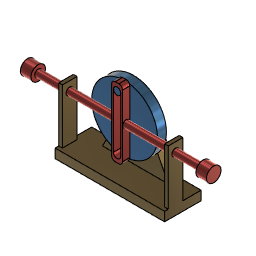
Scotch Yoke Mechanism (Autodesk Fusion 360 design; units mm, degrees)
Autodesk Fusion 360 part; units mm, degrees
sketch "Holder Base" plane through (0, 0, 0) normal (0, 0, 1) x (1, 0, 0)
  line L0 (150, -50) -> (-150, -50)
  line L1 (-150, -50) -> (-150, 50)
  line L2 (-150, 50) -> (150, 50)
  line L3 (150, 50) -> (150, -50)
  line L4 (150, -50) -> (-150, 50) construction
  line L5 (-150, -50) -> (150, 50) construction
  dimension "d1" = 300
  dimension "d2" = 100
  constraint horizontal L0
  constraint perpendicular L0 L1
  constraint parallel L0 L2
  constraint parallel L1 L3
  constraint coincident L4 origin
  constraint coincident L5 origin
  measures "d1" distance of L1.end L2.end
  measures "d2" distance of L0.end L1.end
extrude "Extrude1" add sketch "Holder Base" along normal blind 25 makes body 1
sketch "Holder" plane through (0, 0, 25) normal (0, 0, 1) x (-1, 0, 0)
  line L0 (-150, -50) -> (150, -50)
  line L1 (150, -50) -> (150, 50)
  line L2 (150, 50) -> (-150, 50)
  line L3 (-150, 50) -> (-150, -50)
  line L4 (-90, -50) -> (90, -50)
  line L5 (90, -50) -> (90, -20)
  line L6 (90, -20) -> (-90, -20)
  line L7 (-90, -20) -> (-90, -50)
  constraint horizontal L4
  constraint vertical L5
  constraint horizontal L6
  constraint vertical L7
  constraint coincident L0 L4.start
extrude "Extrude2" add sketch "Holder" along normal blind 150 contours L0 L4 L5 L6 L7 bodies 1
sketch "Holder Shape" plane through (0, 20, 0) normal (0, -1, 0) x (1, 0, 0)
  line L0 (-90, 25) -> (90, 25)
  line L1 (90, 25) -> (90, 175)
  line L2 (90, 175) -> (-90, 175)
  line L3 (-90, 175) -> (-90, 25)
  circle A0 centre (0, 150) radius 25
  line L4 (-90, 25) -> (-22.3903, 161.121)
  line L5 (90, 25) -> (22.3903, 161.121)
  circle A1 centre (0, 150) radius 10
  constraint tangent L2 A0
  constraint coincident L0.start L3.end
  constraint coincident A0 L4.end
  constraint tangent A0 L4
  constraint coincident L0.end L1.start
  constraint coincident A0 L5.end
  constraint tangent A0 L5
  constraint concentric A0 A1
extrude "Extrude3" cut sketch "Holder Shape" against normal blind 70 contours L2 L3 A0 L4 | L1 L2 A0 L5 bodies 1
sketch "Crank" plane through (0, 20, 93.0605) normal (0, -1, 0) x (1, 0, 0)
  circle A0 centre (0, 56.9395) radius 90
  point P0 (0, 56.9395)
  dimension "d9" = 180
  constraint coincident P0 A0.centre
  measures "d9" diameter of A0
extrude "Extrude4" add sketch "Crank" along normal blind 30 and the other way blind -10 separate body makes body 2
extrude "Extrude5" cut sketch "Holder Shape" along normal blind 150 contours A1 bodies 2
extrude "Extrude6" add sketch "Holder Shape" along normal blind 4.8 contours A0 bodies 1
extrude "Extrude7" add 1 faces at (62.9983, 10, 145.5287) along direction (0, 1, 0) blind 5 on bodies 2 bodies 2
extrude "Extrude8" add sketch "Holder Shape" along normal blind 40 contours A1 bodies 1
extrude "Extrude9" cut 1 faces at (3.0405, -20, 148.0569) along direction (0, 1, 0) blind 10 on bodies 1 bodies 1
move_face "OffsetFaces1" offset -0.3 1 faces at (9.9876, 6.6667, 150.4985) on bodies 2
move_face "OffsetFaces2" offset -0.3 1 faces at (10.2872, -1.6667, 149.4866) on bodies 2
sketch "Crank Pin" plane through (0, -10, 0) normal (0, -1, 0) x (1, 0, 0)
  circle A0 centre (75, 150) radius 10
extrude "Extrude10" add sketch "Crank Pin" along normal blind 20 bodies 2
sketch "Slotted Link" plane through (0, -10, 0) normal (0, -1, 0) x (1, 0, 0)
  line L0 (75, 235) -> (75, 235)
  line L1 (85, 225) -> (85, 75)
  line L2 (75, 65) -> (75, 65)
  line L3 (65, 75) -> (65, 225)
  line L4 (70, 245) -> (80, 245)
  line L5 (90, 235) -> (90, 64.9408)
  line L6 (80, 54.9408) -> (70, 54.9408)
  line L7 (60, 64.9408) -> (60, 235)
  arc A0 (85, 225) -> (75, 235) centre (75, 225) ccw
  arc A1 (75, 235) -> (65, 225) centre (75, 225) ccw
  arc A2 (90, 235) -> (80, 245) centre (80, 235) ccw
  arc A3 (70, 245) -> (60, 235) centre (70, 235) ccw
  arc A4 (80, 54.9408) -> (90, 64.9408) centre (80, 64.9408) ccw
  arc A5 (60, 64.9408) -> (70, 54.9408) centre (70, 64.9408) ccw
  arc A6 (75, 65) -> (85, 75) centre (75, 75) ccw
  arc A7 (65, 75) -> (75, 65) centre (75, 75) ccw
  dimension "d28" = 10
  dimension "d29" = 10
  dimension "d30" = 10
  dimension "d31" = 10
  constraint vertical L1
  constraint vertical L3
  constraint horizontal L4
  constraint vertical L5
  constraint horizontal L6
  constraint vertical L7
  constraint tangent L1 A0
  constraint tangent L3 A1
  constraint tangent L4 A2
  constraint tangent L5 A2
  constraint tangent L4 A3
  constraint tangent L7 A3
  constraint equal A2 A3
  constraint tangent L5 A4
  constraint tangent L6 A4
  constraint equal A2 A4
  constraint tangent L6 A5
  constraint tangent L7 A5
  constraint equal A2 A5
  constraint tangent L1 A6
  constraint equal A2 A6
  constraint tangent L3 A7
  measures "d28" radius of A0
  measures "d29" radius of A1
  measures "d30" radius of A2
  measures "d31" radius of A7
extrude "Extrude11" add sketch "Slotted Link" along normal blind 20 separate body makes body 3
extrude "Extrude12" cut 1 faces at (47.1382, -10, 124.9243) along direction (0, 1, 0) blind 0.3 on bodies 2 bodies 2
move_face "OffsetFaces3" offset -0.3 1 faces at (84.9876, -16.4667, 149.5015) on bodies 2
sketch "Piston Holders" plane through (0, 0, 25) normal (0, 0, 1) x (-1, 0, 0)
  line L0 (90, -20) -> (90, -50)
  line L1 (90, -50) -> (150, -50)
  line L2 (150, -50) -> (150, 50)
  line L3 (150, 50) -> (-150, 50)
  line L4 (-150, 50) -> (-150, -50)
  line L5 (-150, -50) -> (-90, -50)
  line L6 (-90, -50) -> (-90, -20)
  line L7 (-90, -20) -> (90, -20)
  line L8 (140, 0) -> (150, 0)
  line L9 (150, 0) -> (150, 40)
  line L10 (150, 40) -> (140, 40)
  line L11 (140, 40) -> (140, 0)
  line L12 (-150, 0) -> (-140, 0)
  line L13 (-140, 0) -> (-140, 40)
  line L14 (-140, 40) -> (-150, 40)
  line L15 (-150, 40) -> (-150, 0)
  constraint horizontal L8
  constraint vertical L9
  constraint horizontal L10
  constraint vertical L11
  constraint coincident L2 L9.end
  constraint horizontal L12
  constraint vertical L13
  constraint horizontal L14
  constraint vertical L15
  constraint midpoint L4 L12.start
extrude "Extrude13" add sketch "Piston Holders" along normal blind 150 contours L2 L8 L9 L10 L11 | L4 L12 L13 L14 L15 bodies 1
sketch "Right Piston" plane through (90, 0, 0) normal (1, 0, 0) x (0, 1, 0)
  line L0 (-10, 64.9408) -> (-10, 235)
  line L1 (-10, 235) -> (-30, 235)
  line L2 (-30, 235) -> (-30, 64.9408)
  line L3 (-30, 64.9408) -> (-10, 64.9408)
  circle A0 centre (-20, 150) radius 10
  constraint tangent L2 A0
sketch "Left Piston" plane through (60, 0, 0) normal (-1, 0, 0) x (0, -1, 0)
  line L0 (10, 235) -> (10, 64.9408)
  line L1 (10, 64.9408) -> (30, 64.9408)
  line L2 (30, 64.9408) -> (30, 235)
  line L3 (30, 235) -> (10, 235)
  circle A0 centre (20, 150) radius 10
extrude "Extrude14" cut sketch "Right Piston" along normal blind 75 contours A0 bodies 1
extrude "Extrude15" cut sketch "Left Piston" along normal blind 230 contours A0 bodies 1
extrude "Extrude16" add sketch "Left Piston" along normal blind 240 contours A0 bodies 3
extrude "Extrude17" add sketch "Right Piston" along normal blind 240 contours A0 bodies 3
sketch "Left Piston End" plane through (-180, 0, 0) normal (-1, 0, 0) x (0, -1, 0)
  circle A0 centre (20, 150) radius 10
  circle A1 centre (20, 150) radius 20
  constraint concentric A0 A1
extrude "Extrude18" add sketch "Left Piston End" against normal blind 29 bodies 3
sketch "Right Piston End" plane through (330, 0, 0) normal (1, 0, 0) x (0, 1, 0)
  circle A0 centre (-20, 150) radius 10
  circle A1 centre (-20, 150) radius 20
  dimension "d49" = 40
  constraint concentric A0 A1
  measures "d49" diameter of A1
extrude "Extrude19" add sketch "Right Piston End" against normal blind 29 bodies 3
move_face "OffsetFaces4" offset -0.3 2 faces at (160.3333, -10.0497, 149.0043) (-80.6667, -29.9876, 149.5015) on bodies 3
copy_body "Body->Comp1" bodies 1 removing the originals makes body 4 in component "Holder"
copy_body "Body->Comp2" bodies 2 removing the originals makes body 5 in component "Crank"
copy_body "Body->Comp3" bodies 3 removing the originals makes body 6 in component "Slotted Link"
component "Holder" placed x (1, 0, 0) y (0, 1, 0) z (0, 0, 1) at (0, 0, 0)
component "Crank" placed x (1, 0, 0) y (0, 1, 0) z (0, 0, 1) at (0, 0, 0)
component "Slotted Link" placed x (1, 0, 0) y (0, 1, 0) z (0, 0, 1) at (0, 0, 0)
named bodies: "Holder", "Crank", "Slotted Link"
